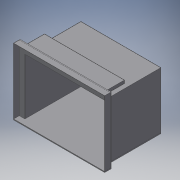
# Autodesk Inventor part: Tank2
Saved by Autodesk Inventor 2019 (Build 230136000, 136)
## iProperties
Created: 2020-03-11
Part Number: Tank2
Material: Generic
Document SubType Name: Modeling
Designer: Vijay
Density: 1 g/cm^3
Appearance: Default
Author: Vijay
Autodesk Inventor part; units mm, degrees
ref_plane "YZ Plane" through (0, 0, 0) normal (1, 0, 0) x (0, 1, 0)
ref_plane "XZ Plane" through (0, 0, 0) normal (0, 1, 0) x (-1, 0, 0)
ref_plane "XY Plane" through (0, 0, 0) normal (0, 0, 1) x (1, 0, 0)
sketch "Sketch1" plane through (0, 0, 0) normal (0, 0, 1) x (1, 0, 0)
  line L0 (-204, -167.1829) -> (204, -167.1829) construction
  line L1 (204, -167.1829) -> (204, 115) construction
  line L2 (204, 115) -> (-204, 115) construction
  line L3 (-204, 115) -> (-204, -167.1829) construction
  line L4 (-214, -177.1829) -> (214, -177.1829)
  line L5 (214, -177.1829) -> (214, 125)
  line L6 (214, 125) -> (-214, 125)
  line L7 (-214, 125) -> (-214, -177.1829)
  line L8 (-244, -177.1829) -> (244, -177.1829)
  line L9 (244, -177.1829) -> (244, 175)
  line L10 (244, 175) -> (-244, 175)
  line L11 (-244, 175) -> (-244, -177.1829)
  point P0 (0, 0)
  dimension "d0" = 10
  dimension "d1" = 30
  dimension "d2" = 30
  dimension "d3" = 50
  constraints: 24 end point, 6 parallel, 3 perpendicular, 2 horizontal, 5 other
  measures "d0" distance between parallel lines of L3 L7
  measures "d1" distance between parallel lines of L7 L11
  measures "d2" distance between parallel lines of L9 L5
  measures "d3" distance between parallel lines of L6 L10
extrude "Extrusion1" add sketch "Sketch1" along normal blind 5 contours L8 L11 L10 L9 L5 L6 L7
sketch "Sketch2" plane through (0, 0, 5) normal (0, 0, 1) x (1, 0, 0)
  line L0 (-214, -177.1829) -> (-214, 125) projected
  line L1 (-214, 125) -> (214, 125) projected
  line L2 (214, 125) -> (214, -177.1829) projected
  line L3 (214, -177.1829) -> (244, -177.1829) projected
  line L4 (244, -177.1829) -> (244, 175) projected
  line L5 (244, 175) -> (-244, 175) projected
  line L6 (-244, 175) -> (-244, -177.1829) projected
  line L7 (-244, -177.1829) -> (-214, -177.1829) projected
  line L8 (213.2, 124.2) -> (-213.2, 124.2)
  line L9 (-213.2, 124.2) -> (-213.2, -176.3829)
  line L10 (-244, -177.9829) -> (-244.8, -177.9829)
  line L11 (-244.8, -177.9829) -> (-244.8, 175.8)
  line L12 (-244.8, 175.8) -> (244.8, 175.8)
  line L13 (244.8, 175.8) -> (244.8, -177.9829)
  line L14 (244.8, -177.9829) -> (213.2, -177.9829)
  line L15 (214, 125) -> (214, -177.1829) projected
  line L16 (-244, -177.1829) -> (-214, -177.1829) projected
  line L17 (213.2, -177.1829) -> (-214, -177.1829)
  line L18 (213.2, -176.3829) -> (-213.2, -176.3829)
  line L19 (213.2, -177.1829) -> (214, -177.1829)
  line L20 (213.2, -177.9829) -> (213.2, -177.1829)
  line L21 (213.2, -176.3829) -> (213.2, 124.2)
  point P0 (0, 0)
  dimension "d6" = 0.8
  dimension "d7" = 0.8
  constraints: 24 end point, 2 horizontal, 1 perpendicular, 1 point on line, 3 other
  measures "d6" distance between parallel lines of L3 L14
  measures "d7" distance between parallel lines of L18 L17
extrude "Extrusion2" add sketch "Sketch2" against normal blind 300 contours L0 L1 L2 L19 L17
sketch "Sketch3" plane through (0, 0, 5) normal (0, 0, 1) x (1, 0, 0)
  line L0 (-213.2, -176.3829) -> (-213.2, 124.2) projected
  line L1 (-213.2, 124.2) -> (213.2, 124.2) projected
  line L2 (213.2, 124.2) -> (213.2, -176.3829) projected
  line L3 (213.2, -176.3829) -> (-213.2, -176.3829) projected
  line L4 (-244, -177.1829) -> (244, -177.1829) projected
  line L5 (244, -177.1829) -> (244, 175) projected
  line L6 (244, 175) -> (-244, 175) projected
  line L7 (-244, 175) -> (-244, -177.1829) projected
  line L8 (243.2, -176.3829) -> (-243.2, -176.3829)
  line L9 (-243.2, -176.3829) -> (-243.2, 174.2)
  line L10 (-243.2, 174.2) -> (243.2, 174.2)
  line L11 (243.2, 174.2) -> (243.2, -176.3829)
  point P0 (0, 0)
  dimension "d10" = 0.8
  constraints: 8 end point, 3 other
  measures "d10" distance between parallel lines of L4 L8
extrude "Extrusion3" add sketch "Sketch3" along normal blind 30
sketch "Sketch4" plane through (0, 0, 5) normal (0, 0, 1) x (1, 0, 0)
  line L0 (-213.2, 156.7) -> (213.2, 156.7) construction
  line L1 (-213.2, 164.2) -> (213.2, 164.2)
  line L2 (213.2, 149.2) -> (-213.2, 149.2)
  line L3 (-213.2, -176.3829) -> (-213.2, 124.2) projected
  line L4 (213.2, 124.2) -> (213.2, -176.3829) projected
  line L5 (-243.2, 174.2) -> (243.2, 174.2) projected
  line L6 (213.2, 164.2) -> (213.2, 149.2)
  line L7 (-213.2, 124.2) -> (213.2, 124.2) projected
  line L8 (-213.2, 149.2) -> (-213.2, 164.2)
  point P0 (0, 0)
  point P1 (0, 156.7)
  dimension "d13" = 15
  dimension "d14" = 10
  constraints: 12 end point, 2 parallel, 2 point on line, 1 horizontal, 1 midpoint, 1 perpendicular
  measures "d13" distance between parallel lines of L2 L1
  measures "d14" distance between parallel lines of L5 L1
extrude "Extrusion4" cut sketch "Sketch4" against normal blind 30
sketch "Sketch5" plane through (0, 0, -295) normal (0, 0, -1) x (-1, 0, 0)
  line L0 (213.2, 124.2) -> (213.2, -176.3829) projected
  line L1 (213.2, -176.3829) -> (-213.2, -176.3829) projected
  line L2 (-213.2, -176.3829) -> (-213.2, 124.2) projected
  line L3 (-213.2, 124.2) -> (213.2, 124.2) projected
  line L4 (-214, -177.1829) -> (214, -177.1829) projected
  line L5 (214, -177.1829) -> (214, 125) projected
  line L6 (214, 125) -> (-214, 125) projected
  line L7 (-214, 125) -> (-214, -177.1829) projected
  point P0 (0, 0)
extrude "Extrusion5" add sketch "Sketch5" along normal blind 0.8 contours L0 L1 L2 L3 | L7 L6 L5 L4
sketch "Sketch6" plane through (0, 0, 0) normal (0, 0, -1) x (-1, 0, 0)
  line L0 (213.2, 164.2) -> (213.2, 149.2) projected
  line L1 (213.2, 149.2) -> (-213.2, 149.2) projected
  line L2 (-213.2, 149.2) -> (-213.2, 164.2) projected
  line L3 (-213.2, 164.2) -> (213.2, 164.2) projected
  line L4 (214, 125) -> (214, -177.1829) projected
  line L5 (244, -177.1829) -> (214, -177.1829) projected
  line L6 (244, 175) -> (244, -177.1829) projected
  line L7 (-244, 175) -> (244, 175) projected
  line L8 (-244, -177.1829) -> (-244, 175) projected
  line L9 (-214, -177.1829) -> (-244, -177.1829) projected
  line L10 (-214, -177.1829) -> (-214, 125) projected
  line L11 (-214, 125) -> (214, 125) projected
  line L12 (-214, 148.4) -> (214, 148.4)
  line L13 (214, 148.4) -> (214, 165)
  line L14 (214, 165) -> (-214, 165)
  line L15 (-214, 165) -> (-214, 148.4)
  point P0 (0, 0)
  dimension "d19" = 0.8
  constraints: 8 end point, 3 other
  measures "d19" distance between parallel lines of L1 L12
extrude "Extrusion6" add sketch "Sketch6" along normal blind 100 contours L15 L14 L13 L12
sketch "Sketch7" plane through (214, -177.1829, 0) normal (0, -1, 0) x (1, 0, 0)
  line L0 (0, 0) -> (30, 0) projected
  line L1 (30, 0) -> (30, 35) projected
  line L2 (-458, 35) -> (30, 35) projected
  line L3 (-458, 0) -> (-458, 35) projected
  line L4 (-458, 0) -> (-428, 0) projected
  line L5 (-428, 0) -> (-428, -295.8) projected
  line L6 (0, -295.8) -> (-428, -295.8) projected
  line L7 (0, 0) -> (0, -295.8) projected
  point P0 (-214, 0)
extrude "Extrusion7" add sketch "Sketch7" along normal blind 4.2
sketch "Sketch8" plane through (0, 0, -100) normal (0, 0, -1) x (-1, 0, 0)
  line L0 (213.2, 149.2) -> (-213.2, 149.2) projected
  line L1 (-213.2, 149.2) -> (-213.2, 164.2) projected
  line L2 (-213.2, 164.2) -> (213.2, 164.2) projected
  line L3 (213.2, 164.2) -> (213.2, 149.2) projected
  line L4 (-214, 148.4) -> (214, 148.4) projected
  line L5 (214, 148.4) -> (214, 165) projected
  line L6 (214, 165) -> (-214, 165) projected
  line L7 (-214, 165) -> (-214, 148.4) projected
  point P0 (0, 0)
extrude "Extrusion8" add sketch "Sketch8" along normal blind 0.8 contours L0 L1 L2 L3 | L7 L6 L5 L4
sketch "Sketch9" plane through (0, 0, -100.8) normal (0, 0, -1) x (-1, 0, 0)
  line L0 (-213.2, 164.2) -> (-213.2, 149.2) construction
  line L1 (-213.2, 156.7) -> (441.8392, 156.7) construction
  circle A0 centre (0, 156.7) radius 5
  point P0 (0, 0)
  dimension "d26" = 10
  constraints: 2 end point, 1 centre point, 1 horizontal, 1 midpoint, 1 point on line
  measures "d26" diameter of A0
extrude "Extrusion9" cut sketch "Sketch9" against normal blind 0.8
sketch "Sketch10" plane through (-214, 125, 0) normal (0, 1, 0) x (1, 0, 0)
  line L0 (428, 0) -> (0, 0) projected
  line L1 (428, 0) -> (428, 295.8) projected
  line L2 (0, 295.8) -> (428, 295.8) projected
  line L3 (0, 0) -> (0, 295.8) projected
  point P0 (214, 0)
extrude "Extrusion10" add sketch "Sketch10" along normal blind 4.2
body "Solid1"
